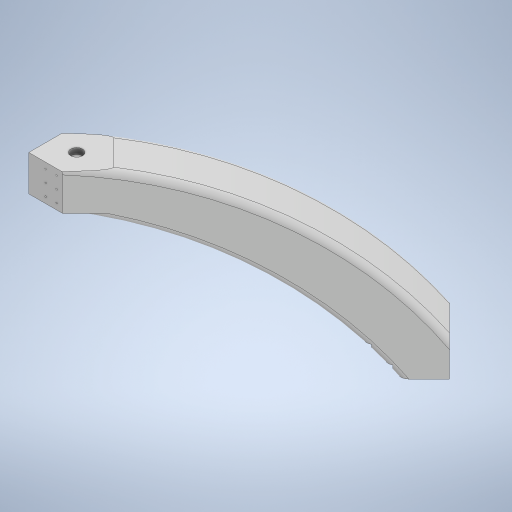
# Autodesk Inventor part: Table Leg X4
Saved by Autodesk Inventor 2023 (Build 270158000, 158)
## iProperties
Created: 2022-11-22
Part Number: Table Leg X4
Material: Generic
Document SubType Name: Modeling
Designer: surat
Density: 1 g/cm^3
Appearance: Default
Author: surat
Autodesk Inventor part; units mm, degrees
ref_plane "YZ Plane" through (0, 0, 0) normal (1, 0, 0) x (0, 1, 0)
ref_plane "XZ Plane" through (0, 0, 0) normal (0, 1, 0) x (-1, 0, 0)
ref_plane "XY Plane" through (0, 0, 0) normal (0, 0, 1) x (1, 0, 0)
sketch "Sketch1" plane through (0, 0, 0) normal (0, 1, 0) x (-1, 0, 0)
  line L0 (6.35, 0) -> (1365.25, 0)
  line L1 (1371.6, -6.35) -> (1371.6, -1365.25)
  line L2 (1365.25, -1371.6) -> (6.35, -1371.6)
  line L3 (0, -1365.25) -> (0, -6.35)
  line L4 (1346.2, -1346.2) -> (1346.2, -25.4)
  line L5 (1346.2, -25.4) -> (25.4, -25.4)
  line L6 (25.4, -25.4) -> (25.4, -1346.2)
  line L7 (25.4, -1346.2) -> (1346.2, -1346.2)
  line L8 (1320.8, -50.8) -> (1320.8, -1320.8)
  line L9 (1320.8, -1320.8) -> (50.8, -1320.8)
  line L10 (50.8, -1320.8) -> (50.8, -50.8)
  line L11 (50.8, -50.8) -> (1320.8, -50.8)
  line L12 (1320.8, -50.8) -> (1346.2, -25.4)
  line L13 (1320.8, -1320.8) -> (1346.2, -1346.2)
  line L14 (50.8, -1320.8) -> (25.4, -1346.2)
  line L15 (50.8, -50.8) -> (25.4, -25.4)
  line L16 (1365.25, 0) -> (1371.6, -6.35)
  line L17 (1371.6, -1365.25) -> (1365.25, -1371.6)
  line L18 (6.35, -1371.6) -> (0, -1365.25)
  line L19 (6.35, 0) -> (0, -6.35)
  line L20 (1320.8, -50.8) -> (50.8, -1320.8)
  line L21 (1320.8, -1320.8) -> (50.8, -50.8)
  line L22 (1320.8, -122.642) -> (122.642, -1320.8)
  line L23 (50.8, -1248.958) -> (1248.958, -50.8)
  line L24 (50.8, -122.642) -> (1248.958, -1320.8)
  line L25 (1320.8, -1248.958) -> (122.642, -50.8)
  line L26 (910.042, -533.4) -> (910.042, -838.2)
  line L27 (838.2, -910.042) -> (533.4, -910.042)
  line L28 (461.558, -838.2) -> (461.558, -533.4)
  line L29 (838.2, -461.558) -> (533.4, -461.558)
  line L30 (838.2, -461.558) -> (910.042, -533.4)
  line L31 (910.042, -838.2) -> (838.2, -910.042)
  line L32 (533.4, -910.042) -> (461.558, -838.2)
  line L33 (461.558, -533.4) -> (533.4, -461.558)
  arc A0 (910.042, -533.4) -> (910.042, -838.2) centre (1259.2343, -685.8) ccw
  arc A1 (838.2, -910.042) -> (533.4, -910.042) centre (685.8, -1259.2343) ccw
  arc A2 (461.558, -838.2) -> (461.558, -533.4) centre (112.3657, -685.8) ccw
  arc A3 (533.4, -461.558) -> (838.2, -461.558) centre (685.8, -112.3657) ccw
  point P0 (0, 0)
  point P1 (1371.6, -1371.6)
  point P2 (1371.6, 0)
  point P3 (0, -1371.6)
  dimension "d0" = 1371.6
  dimension "d1" = 1371.6
  dimension "d2" = 25.4
  dimension "d3" = 25.4
  dimension "d34" = 6.35
  dimension "d35" = 6.35
  dimension "d36" = 6.35
  dimension "d37" = 6.35
  dimension "d38" = 6.35
  dimension "d39" = 6.35
  dimension "d40" = 6.35
  dimension "d41" = 6.35
  dimension "d42" = 50.8
  dimension "d43" = 50.8
  dimension "d44" = 50.8
  dimension "d45" = 50.8
  dimension "d46" = 304.8
  dimension "d47" = 304.8
  dimension "d48" = 304.8
  dimension "d50" = 304.8
  dimension "d51" = 381
  dimension "d52" = 381
  dimension "d53" = 381
  dimension "d54" = 381
  constraints: 68 end point, 26 point on line, 10 parallel, 10 perpendicular, 8 point on circle, 4 centre point, 2 horizontal, 1 vertical, 6 other
  measures "d0" distance of point (1371.6, -1371.6) point (0, -1371.6)
  measures "d1" distance of point (1371.6, 0) point (1371.6, -1371.6)
  measures "d2" distance between parallel lines of L1 L4
  measures "d3" distance between parallel lines of L4 L8
  measures "d34" distance of L0.end point (1371.6, 0)
  measures "d35" distance of L1.start point (1371.6, 0)
  measures "d36" distance of L1.end point (1371.6, -1371.6)
  measures "d37" distance of L2.start point (1371.6, -1371.6)
  measures "d38" distance of L2.end point (0, -1371.6)
  measures "d39" distance of L3.start point (0, -1371.6)
  measures "d40" distance of L0.start point (0, 0)
  measures "d41" distance of L3.end point (0, 0)
  measures "d42" distance between parallel lines of L21 L25
  measures "d43" distance between parallel lines of L24 L21
  measures "d44" distance between parallel lines of L23 L20
  measures "d45" distance between parallel lines of L22 L20
  measures "d46" distance of L26.start L26.end
  measures "d47" distance of L27.start L27.end
  measures "d48" distance of L28.start L28.end
  measures "d50" distance of L29.start L29.end
  measures "d51" radius of A0
  measures "d52" radius of A1
  measures "d53" radius of A2
  measures "d54" radius of A3
sketch "Sketch2" plane through (0, 0, 0) normal (0, 1, 0) x (-1, 0, 0)
  point P0 (0, 0)
extrude "Extrusion1" add sketch "Sketch1" along normal blind 381 contours L20 L30 L23 L11 | L8 L22 L30 L20
sketch "Sketch3" plane through (-838.2, 0, -461.558) normal (0.7071, 0, 0.7071) x (0.7071, 0, -0.7071)
  line L0 (0, 0) -> (0, 381) projected
  line L1 (-580.8995, 0) -> (0, 0) projected
  line L2 (0, 76.2) -> (-504.6995, 381)
  line L3 (-580.8995, 381) -> (0, 381) projected
  line L4 (-580.8995, 304.8) -> (-76.2, 0)
  arc A0 (-76.2, 0) -> (-580.8995, 304.8) centre (-691.8017, -449.0864) ccw
  arc A1 (0, 76.2) -> (-504.6995, 381) centre (-615.6017, -372.8864) ccw
  line L5 (-580.8995, 304.8) -> (-849.8669, 304.8)
  line L6 (-849.8669, 304.8) -> (-849.8669, -233.7974)
  line L7 (-849.8669, -233.7974) -> (129.4669, -282.8932)
  line L8 (129.4669, -282.8932) -> (-76.2, 0)
  point P0 (266.3261, 0)
  point P1 (-76.2, 0)
  dimension "d57" = 76.2
  dimension "d58" = 76.2
  dimension "d59" = 76.2
  dimension "d60" = 76.2
  dimension "d61" = 762
  dimension "d62" = 762
  constraints: 12 end point, 4 point on circle, 3 point on line, 2 centre point, 1 horizontal, 1 perpendicular
  measures "d57" distance from line of L1 L2.start
  measures "d58" distance of L3.start L2.end
  measures "d59" distance of L4.start L3.start
  measures "d60" distance of L0.start L4.end
  measures "d61" radius of A0
  measures "d62" radius of A1
extrude "Extrusion2" cut sketch "Sketch3" against normal blind 381 contours A1 L3 L0 | L8 L7 L6 L5 L4 | L4 A0
sketch "Sketch4" plane through (-1320.8, 381, -50.8) normal (0, 0, 1) x (1, 0, 0)
  circle A0 centre (35.9156, -12.7) radius 1.5875
  circle A1 centre (59.142, -12.7) radius 1.5875
  circle A2 centre (59.142, -63.5) radius 1.5875
  circle A3 centre (35.9156, -63.5) radius 1.5875
  circle A4 centre (35.9156, -38.1) radius 1.5875
  line L0 (0, 0) -> (71.842, 0) projected
  line L1 (0, -76.2) -> (0, 0) projected
  line L2 (71.842, -76.2) -> (71.842, 0) projected
  line L3 (0, -76.2) -> (71.842, -76.2) projected
  circle A5 centre (59.142, -38.1) radius 1.5875
  point P0 (1320.8, -381)
  point P1 (0, -38.1)
  dimension "d65" = 3.175
  dimension "d66" = 3.175
  dimension "d67" = 3.175
  dimension "d68" = 3.175
  dimension "d69" = 3.175
  dimension "d70" = 12.7
  dimension "d71" = 35.9156
  dimension "d72" = 12.7
  dimension "d73" = 12.7
  dimension "d74" = 12.7
  dimension "d75" = 12.7
  dimension "d76" = 12.7
  dimension "d77" = 35.9156
  dimension "d78" = 38.1
  dimension "d79" = 35.9156
  dimension "d95" = 3.175
  dimension "d96" = 38.1
  dimension "d97" = 12.7
  constraints: 6 centre point, 1 midpoint
  measures "d65" diameter of A0
  measures "d66" diameter of A1
  measures "d67" diameter of A2
  measures "d68" diameter of A3
  measures "d69" diameter of A4
  measures "d70" distance from line of L0 A0.centre
  measures "d71" distance from line of L1 A0.centre
  measures "d72" distance from line of L0 A1.centre
  measures "d73" distance from line of L2 A1.centre
  measures "d74" distance from line of L2 A2.centre
  measures "d75" distance from line of L3 A2.centre
  measures "d76" distance from line of L3 A3.centre
  measures "d77" distance from line of L1 A3.centre
  measures "d78" distance from line of L0 A4.centre
  measures "d79" distance of point (0, -38.1) A4.centre
  measures "d95" diameter of A5
  measures "d96" distance from line of A5.centre L0
  measures "d97" distance from line of L2 A5.centre
sketch "Sketch5" plane through (-1320.8, 381, -122.642) normal (-1, 0, 0) x (0, 0, 1)
  circle A0 centre (12.7, -12.7) radius 1.5875
  circle A1 centre (35.9264, -12.7) radius 1.5875
  circle A2 centre (12.7, -63.5) radius 1.5875
  circle A3 centre (34.3389, -63.5) radius 1.5875
  line L0 (0, 0) -> (71.842, 0) projected
  line L1 (0, -76.2) -> (0, 0) projected
  line L2 (71.842, -76.2) -> (71.842, 0) projected
  line L3 (0, -76.2) -> (71.842, -76.2) projected
  circle A4 centre (12.7, -38.1) radius 1.5875
  circle A5 centre (35.9264, -38.1) radius 1.5875
  point P0 (122.642, -381)
  dimension "d80" = 3.175
  dimension "d81" = 3.175
  dimension "d83" = 3.175
  dimension "d84" = 3.175
  dimension "d85" = 12.7
  dimension "d86" = 12.7
  dimension "d87" = 12.7
  dimension "d88" = 35.9156
  dimension "d91" = 12.7
  dimension "d92" = 12.7
  dimension "d93" = 12.7
  dimension "d94" = 35.9156
  dimension "d98" = 3.175
  dimension "d99" = 3.175
  dimension "d100" = 35.9156
  dimension "d101" = 38.1
  dimension "d102" = 38.1
  dimension "d103" = 12.7
  constraints: 6 centre point
  measures "d80" diameter of A0
  measures "d81" diameter of A1
  measures "d83" diameter of A2
  measures "d84" diameter of A3
  measures "d85" distance from line of L0 A0.centre
  measures "d86" distance from line of L1 A0.centre
  measures "d87" distance from line of L0 A1.centre
  measures "d88" distance from line of L2 A1.centre
  measures "d91" distance from line of L1 A2.centre
  measures "d92" distance from line of L3 A2.centre
  measures "d93" distance from line of L3 A3.centre
  measures "d94" distance edge to line of A3 L2
  measures "d98" diameter of A4
  measures "d99" diameter of A5
  measures "d100" distance from line of L2 A5.centre
  measures "d101" distance from line of L0 A5.centre
  measures "d102" distance from line of L0 A4.centre
  measures "d103" distance from line of L1 A4.centre
extrude "Extrusion3" cut sketch "Sketch5" against normal blind 25.4 contours A0 | A1 | A2 | A3 | A4 | A5
extrude "Extrusion4" cut sketch "Sketch4" against normal blind 25.4 contours A0 | A1 | A2 | A3 | A4 | A5
sketch "Sketch6" plane through (-838.2, 0, -461.558) normal (0.7071, 0, -0.7071) x (-0.7071, 0, -0.7071)
  circle A0 centre (19.05, 57.15) radius 3.175
  circle A1 centre (19.05, 19.05) radius 3.175
  circle A2 centre (82.55, 57.15) radius 3.175
  circle A3 centre (82.55, 19.05) radius 3.175
  circle A4 centre (50.8, 57.15) radius 3.175
  circle A5 centre (50.8, 19.05) radius 3.175
  line L0 (0, 0) -> (0, 76.2) projected
  line L1 (101.6, 0) -> (101.6, 76.2) projected
  line L2 (101.6, 76.2) -> (0, 76.2) projected
  line L3 (0, 0) -> (101.6, 0) projected
  point P0 (-919.0677, 0)
  point P1 (101.6, 38.1)
  dimension "d108" = 6.35
  dimension "d109" = 6.35
  dimension "d110" = 6.35
  dimension "d111" = 6.35
  dimension "d112" = 6.35
  dimension "d113" = 6.35
  dimension "d114" = 19.05
  dimension "d115" = 19.05
  dimension "d116" = 50.8
  dimension "d117" = 19.05
  dimension "d118" = 19.05
  dimension "d119" = 19.05
  dimension "d120" = 19.05
  dimension "d121" = 19.05
  dimension "d122" = 50.8
  dimension "d123" = 19.05
  dimension "d124" = 19.05
  dimension "d125" = 19.05
  constraints: 6 centre point, 1 midpoint
  measures "d108" diameter of A0
  measures "d109" diameter of A1
  measures "d110" diameter of A2
  measures "d111" diameter of A3
  measures "d112" diameter of A4
  measures "d113" diameter of A5
  measures "d114" distance from line of A0.centre L0
  measures "d115" distance from line of L1 A2.centre
  measures "d116" distance from line of L1 A4.centre
  measures "d117" distance from line of L2 A0.centre
  measures "d118" distance from line of L2 A4.centre
  measures "d119" distance from line of L2 A2.centre
  measures "d120" distance from line of L0 A1.centre
  measures "d121" distance from line of L1 A3.centre
  measures "d122" horizontal distance of point (101.6, 38.1) A5.centre
  measures "d123" distance from line of L3 A1.centre
  measures "d124" distance from line of L3 A5.centre
  measures "d125" distance from line of L3 A3.centre
extrude "Extrusion5" cut sketch "Sketch6" against normal blind 254 contours A0 | A1 | A2 | A3 | A4 | A5
fillet "Fillet1" radius 12.7 4 edges at (-994.9483, 279.3914, -304.8096) (-1048.8299, 203.1914, -250.9281) (-1066.7904, 279.3914, -376.6517) (-1120.6719, 203.1914, -322.7701)
sketch "Sketch7" plane through (-1248.958, 304.8, -50.8) normal (0.7071, 0, 0.7071) x (0.7071, 0, -0.7071)
  line L0 (445.0278, -241.3) -> (463.8885, -241.3)
  line L1 (463.8885, -241.3) -> (463.8885, -260.6442)
  line L2 (463.8885, -260.6442) -> (445.0278, -260.6442)
  line L3 (445.0278, -260.6442) -> (445.0278, -241.3)
  line L4 (475.1524, -279.4) -> (495.7262, -279.4)
  line L5 (495.7262, -279.4) -> (495.7262, -300.6902)
  line L6 (495.7262, -300.6902) -> (475.1524, -300.6902)
  line L7 (475.1524, -300.6902) -> (475.1524, -279.4)
  line L8 (1590.2918, -247.65) -> (-394.4345, -247.65) projected
  line L9 (1590.2918, -285.75) -> (-394.4345, -285.75) projected
  arc A0 (504.6995, -304.8) -> (0, 0) centre (-110.9022, -753.8864) ccw projected
  point P0 (847.2256, -304.8)
  dimension "d129" = 6.35
  dimension "d130" = 6.35
  constraints: 16 end point, 4 parallel, 2 horizontal, 2 perpendicular
  measures "d129" distance between parallel lines of L0 L8
  measures "d130" distance between parallel lines of L9 L4
extrude "Extrusion6" cut sketch "Sketch7" against normal blind 254
sketch "Sketch8" plane through (0, 381, 0) normal (0, 1, 0) x (1, 0, 0)
  circle A0 centre (-1270, 101.6) radius 3.175
  line L0 (-1320.8, 122.642) -> (-910.042, 533.4) projected
  line L1 (-1320.8, 120.9827) -> (-1320.8, 50.8) projected
  circle A1 centre (-1270, 101.6) radius 12.7
  point P0 (0, 0)
  dimension "d133" = 6.35
  dimension "d134" = 50.8
  dimension "d135" = 50.8
  dimension "d136" = 25.4
  constraints: 2 centre point, 1 coincident
  measures "d133" diameter of A0
  measures "d134" distance from line of A0.centre L0
  measures "d135" distance from line of L1 A0.centre
  measures "d136" diameter of A1
extrude "Extrusion7" cut sketch "Sketch8" against normal blind 12.446 contours A0 | A1
sketch "Sketch9" plane through (-1270, 368.554, -101.6) normal (0, 1, 0) x (1, 0, 0)
  circle A0 centre (0, 0) radius 3.175
  point P0 (1270, -101.6)
  dimension "d139" = 6.35
  constraints: 1 centre point
  measures "d139" diameter of A0
extrude "Extrusion8" cut sketch "Sketch9" against normal blind 76.2
hole "Hole1" at (-1270, 301.4033, -101.6) direction (0, -1, 0) diameter 25.4 depth 25.4
hole "Hole2" at (-1270, 301.4033, -101.6) direction (0, 1, 0) diameter 25.4 depth 25.4
equation "\"d35\" = d34"
equation "\"d36\" = d34"
equation "\"d37\" = d36"
equation "\"d38\" = d34"
equation "\"d39\" = d38"
equation "\"d40\" = d34"
equation "\"d41\" = d40"
body "Solid1"
